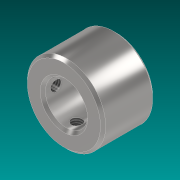
# Autodesk Inventor part: koppelstukje nema23
Saved by Autodesk Inventor 2020.2 (Build 242310000, 310)
## iProperties
Created: 2020-05-18
Part Number: koppelstukje nema23
Material: Stainless Steel
Document SubType Name: Modeling
Designer: Svend
Density: 8 g/cm^3
Appearance: Semi-Polished
Author: Svend
Autodesk Inventor part; units mm, degrees
ref_plane "YZ Plane" through (0, 0, 0) normal (1, 0, 0) x (0, 1, 0)
ref_plane "XZ Plane" through (0, 0, 0) normal (0, 1, 0) x (-1, 0, 0)
ref_plane "XY Plane" through (0, 0, 0) normal (0, 0, 1) x (1, 0, 0)
sketch "Sketch1" plane through (0, 0, 0) normal (0, 0, 1) x (1, 0, 0)
  circle A0 centre (0, 0) radius 7.5
  circle A1 centre (0, 0) radius 4.05
  dimension "d0" = 15
  dimension "d1" = 8.1
  constraints: 2 centre point, 2 coincident
  measures "d0" diameter of A0
  measures "d1" diameter of A1
extrude "Extrusion1" add sketch "Sketch1" along normal mid plane 10
sketch "Sketch2" plane through (0, 0, 0) normal (1, 0, 0) x (0, 1, 0)
  line L0 (4.05, -5) -> (-4.05, -5) projected
  line L1 (-4.05, 5) -> (4.05, 5) projected
  point P0 (0, 0)
  point P1 (0, 2.5)
  point P2 (0, -2.5)
  dimension "d4" = 2.5
  dimension "d5" = 2.5
  constraints: 2 vertical alignment
  measures "d4" distance from line of L0 point (0, -2.5)
  measures "d5" distance from line of L1 point (0, 2.5)
hole "Hole1" at (0, 0, 2.5) at (0, 0, -2.5) direction (-1, 0, 0) diameter 2.013 end through all thread size "M2.5x0.45" class "6H" standard "ISO Metric profile"
chamfer "Chamfer1" distance 0.5 angle 45 4 edges at (-7.5, 0, -5) (-7.5, 0, 5) (-4.05, 0, -5) (-4.05, 0, 5)
sketch "Sketch3" plane through (0, 0, 0) normal (0, 1, 0) x (-1, 0, 0)
  line L0 (4.55, 5) -> (-4.55, 5) projected
  line L1 (-4.55, -5) -> (4.55, -5) projected
  point P0 (0, 0)
  point P1 (0, 2.5)
  point P2 (0, -2.5)
  dimension "d19" = 2.5
  dimension "d20" = 2.5
  constraints: 2 vertical alignment
  measures "d19" distance from line of L0 point (0, 2.5)
  measures "d20" distance from line of L1 point (0, -2.5)
hole "Hole2" at (0, 0, 2.5) at (0, 0, -2.5) direction (0, -1, 0) diameter 2.013 end through all thread size "M2.5x0.45" class "6H" standard "ISO Metric profile"
chamfer "Chamfer3" distance 0.3 angle 45 4 edges at (-0.0805, -7.4996, -3.5033) (-0.0805, -7.4996, 1.4967) (-7.5, 0.002, 3.5065) (-7.5, 0.002, -1.4935)
equation "\"d5\" = d4"
equation "\"d20\" = d19"
body "Solid1"
